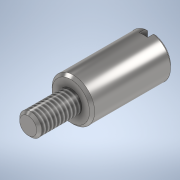
# Autodesk Inventor part: BRU-2609.5S
Saved by Autodesk Inventor 2020.4 (Build 244396000, 396)
## iProperties
Part Number: BRU-2609.5S
Material: ステンレス鋼 AISI 304
Document SubType Name: Modeling
Designer: Masato Kubotera
Density: 7.22596 g/cm^3
Appearance: 半つや出し
Catalog Web Link: https://www.hirosugi-net.co.jp/shop/g/g8609/
Description: ReadyMade
Mass: 1.3165 g
Surface Area: 2.62821 cm^2
Volume: 0.18219 cm^3
Author: Masato Kubotera
Autodesk Inventor part; units mm, degrees
ref_plane "YZ Plane" through (0, 0, 0) normal (1, 0, 0) x (0, 1, 0)
ref_plane "XZ Plane" through (0, 0, 0) normal (0, 1, 0) x (-1, 0, 0)
ref_plane "XY Plane" through (0, 0, 0) normal (0, 0, 1) x (1, 0, 0)
sketch "スケッチ1" plane through (0, 0, 0) normal (0, 1, 0) x (-1, 0, 0)
  line L0 (-1.6, 0) -> (-2.2, 0)
  line L1 (-2.5, 0.3) -> (-2.5, 9.2)
  line L2 (-2.2, 9.5) -> (-1.3, 9.5)
  line L3 (-1.3, 9.5) -> (-1.3, 14.2)
  line L4 (-1, 14.5) -> (0, 14.5)
  line L5 (0, 14.5) -> (0, 5)
  line L6 (0, 5) -> (-1.3, 5)
  line L7 (-1.3, 5) -> (-1.3, 0.3)
  line L8 (-1.3, 14.2) -> (-1, 14.5)
  line L9 (-2.5, 9.2) -> (-2.2, 9.5)
  line L10 (-2.5, 0.3) -> (-2.2, 0)
  line L11 (-1.6, 0) -> (-1.3, 0.3)
  line L12 (0, -2.9) -> (0, 17.4) projected
  point P0 (0, 0)
  point P1 (-2.5, 0)
  point P2 (-2.5, 9.5)
  point P3 (-1.3, 14.5)
  point P4 (-1.3, 0)
  dimension "d0" = 2.6
  dimension "d1" = 5
  dimension "d2" = 9.5
  dimension "d3" = 5
  dimension "d4" = 5
  dimension "d5" = 2.6
  dimension "d6" = 0.3
  dimension "d7" = 0.3
  dimension "d8" = 0.3
  dimension "d9" = 0.3
  dimension "d10" = 0.3
  dimension "d11" = 0.3
  dimension "d12" = 0.3
  dimension "d13" = 0.3
  constraints: 24 end point, 11 point on line, 6 perpendicular, 1 horizontal, 1 parallel
  measures "d0" diameter of point (-1.3, 14.5) L5
  measures "d1" distance of L2.end point (-1.3, 14.5)
  measures "d2" distance of point (-2.5, 0) point (-2.5, 9.5)
  measures "d3" diameter of point (-2.5, 0) L5
  measures "d4" distance of L6.end point (-1.3, 0)
  measures "d5" diameter of L7 L5
  measures "d6" distance of L3.end point (-1.3, 14.5)
  measures "d7" distance of L4.start point (-1.3, 14.5)
  measures "d8" distance of L1.end point (-2.5, 9.5)
  measures "d9" distance of L2.start point (-2.5, 9.5)
  measures "d10" distance of L1.start point (-2.5, 0)
  measures "d11" distance of L0.end point (-2.5, 0)
  measures "d12" distance of L0.start point (-1.3, 0)
  measures "d13" distance of L7.end point (-1.3, 0)
revolve "回転1" add sketch "スケッチ1" angle 360 about axis through (0, 0, -10) along (0, 0, 1)
thread "ねじ1" size "M2.6x0.45" class "6g" standard "ANSI Metric M Profile" full length
thread "ねじ2" size "M2.6x0.45" class "6H" standard "ANSI Metric M Profile" full length
sketch "スケッチ2" plane through (0, 0, 0) normal (0, 0, -1) x (-1, 0, 0)
  line L0 (-0.5, 2.5) -> (0.5, 2.5)
  line L1 (0.5, 2.5) -> (0.5, -2.5)
  line L2 (0.5, -2.5) -> (-0.5, -2.5)
  line L3 (-0.5, -2.5) -> (-0.5, 2.5)
  line L4 (-0.5, 2.5) -> (0.5, -2.5) construction
  line L5 (0.5, 2.5) -> (-0.5, -2.5) construction
  circle A0 centre (0, 0) radius 2.5 projected
  point P0 (0.5, 2.4495)
  point P1 (-0.5, 2.4495)
  point P2 (-0.5, -2.4495)
  point P3 (0.5, -2.4495)
  dimension "d19" = 1
  constraints: 12 end point, 2 midpoint, 2 parallel, 1 horizontal, 1 perpendicular, 1 tangent
  measures "d19" distance of L0.start L0.end
extrude "押し出し1" cut sketch "スケッチ2" against normal blind 1 contours A0 L1 L3
equation "\"d7\" = d6"
equation "\"d8\" = d6"
equation "\"d9\" = d8"
equation "\"d10\" = d6"
equation "\"d11\" = d10"
equation "\"d12\" = d6"
equation "\"d13\" = d12"
